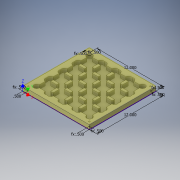
# Autodesk Inventor part: Fixture Glue
Saved by Autodesk Inventor 2016 (Build 200138000, 138)
## iProperties
Created: 2017-01-26
Part Number: Fixture Glue
Material: Generic
Document SubType Name: Modeling
Designer: Samuel Clay
Density: 1 g/cm^3
Appearance: Default
Author: Samuel Clay
Autodesk Inventor part; units mm, degrees
ref_plane "YZ Plane" through (0, 0, 0) normal (1, 0, 0) x (0, 1, 0)
ref_plane "XZ Plane" through (0, 0, 0) normal (0, 1, 0) x (-1, 0, 0)
ref_plane "XY Plane" through (0, 0, 0) normal (0, 0, 1) x (1, 0, 0)
sketch "Sketch1" plane through (0, 0, 0) normal (0, 1, 0) x (-1, 0, 0)
  line L0 (0, 0) -> (-304.8, 0)
  line L1 (-304.8, 0) -> (-304.8, -304.8)
  line L2 (-304.8, -304.8) -> (0, -304.8)
  line L3 (0, -304.8) -> (0, 0)
  point P0 (-12.7, -12.7)
  point P1 (-292.1, -12.7)
  point P2 (-12.7, -292.1)
  point P3 (-292.1, -292.1)
  dimension "d0" = 304.8
  dimension "d1" = 304.8
  dimension "d13" = 12.7
  dimension "d14" = 12.7
  dimension "d15" = 12.7
  dimension "d16" = 12.7
  dimension "d17" = 12.7
  dimension "d18" = 12.7
  dimension "d19" = 12.7
  dimension "d20" = 12.7
  constraints: 8 end point, 2 parallel, 1 horizontal, 1 perpendicular
  measures "d0" distance of L2.end L1.end
  measures "d1" distance of L1.end L0.end
  measures "d13" distance from line of L0 point (-12.7, -12.7)
  measures "d14" distance from line of L3 point (-12.7, -12.7)
  measures "d15" distance from line of L1 point (-292.1, -12.7)
  measures "d16" distance from line of L0 point (-292.1, -12.7)
  measures "d17" distance from line of L2 point (-292.1, -292.1)
  measures "d18" distance from line of L1 point (-292.1, -292.1)
  measures "d19" distance from line of L2 point (-12.7, -292.1)
  measures "d20" distance from line of L3 point (-12.7, -292.1)
extrude "Extrusion1" add sketch "Sketch1" along normal blind 19.05
sketch "Sketch2" plane through (0, 19.05, 0) normal (0, 1, 0) x (1, 0, 0)
  line L0 (31.75, 31.75) -> (83.566, 31.75)
  line L1 (83.566, 31.75) -> (83.566, 83.566)
  line L2 (83.566, 83.566) -> (31.75, 83.566)
  line L3 (31.75, 83.566) -> (31.75, 31.75)
  line L4 (0, 0) -> (304.8, 0) projected
  line L5 (0, 304.8) -> (0, 0) projected
  circle A0 centre (31.75, 31.75) radius 12.7
  circle A1 centre (31.75, 83.566) radius 12.7
  circle A2 centre (83.566, 83.566) radius 12.7
  circle A3 centre (83.566, 31.75) radius 12.7
  dimension "d25" = 51.816
  dimension "d26" = 51.816
  dimension "d27" = 31.75
  dimension "d28" = 31.75
  dimension "d29" = 25.4
  dimension "d30" = 25.4
  dimension "d31" = 25.4
  dimension "d32" = 25.4
  constraints: 8 end point, 4 centre point, 4 coincident, 2 parallel, 1 horizontal, 1 perpendicular
  measures "d25" distance of L2.end L1.end
  measures "d26" distance of L1.end L0.end
  measures "d27" distance from line of L4 L0.start
  measures "d28" distance from line of L5 L0.start
  measures "d29" diameter of A0
  measures "d30" diameter of A1
  measures "d31" diameter of A2
  measures "d32" diameter of A3
extrude "Extrusion3" cut sketch "Sketch2" against normal blind 17.78
pattern_linear "Rectangular Pattern1" count 4 spacing 63.5 along (0, 0, -1) count 4 spacing 63.5 along (1, 0, 0) of "Extrusion3"
hole "Hole1" at (12.7, 0, -12.7) at (292.1, 0, -12.7) at (12.7, 0, -292.1) at (292.1, 0, -292.1) direction (0, 1, 0) diameter 6.35 end through all
equation "\"d13\" = d14"
equation "\"d15\" = d14"
equation "\"d16\" = d13"
equation "\"d17\" = d14"
equation "\"d18\" = d14"
equation "\"d19\" = d14"
equation "\"d20\" = d14"
equation "\"d28\" = d27"
body "Solid1"
